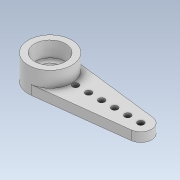
# Autodesk Inventor part: sg90舵盘01
Saved by Autodesk Inventor 2022.5 (Build 265521000, 521)
## iProperties
Created: 2024-03-17
Part Number: sg90舵盘01
Material: 常规
Document SubType Name: Modeling
Designer: Gagouking
Density: 1 g/cm^3
Appearance: 默认
Author: Gagouking
Autodesk Inventor part; units mm, degrees
ref_plane "YZ Plane" through (0, 0, 0) normal (1, 0, 0) x (0, 1, 0)
ref_plane "XZ Plane" through (0, 0, 0) normal (0, 1, 0) x (-1, 0, 0)
ref_plane "XY Plane" through (0, 0, 0) normal (0, 0, 1) x (1, 0, 0)
sketch "草图1" plane through (0, 0, 0) normal (0, 1, 0) x (-1, 0, 0)
  circle A0 centre (0, 0) radius 1.5
  line L0 (0, 0) -> (-13.1253, 0) construction
  circle A1 centre (-4.1, 0) radius 0.5
  circle A2 centre (-6.2, 0) radius 0.5
  circle A3 centre (-8.3, 0) radius 0.5
  circle A4 centre (-10.4, 0) radius 0.5
  circle A5 centre (-12.5, 0) radius 0.5
  circle A6 centre (-14.6, 0) radius 0.5
  arc A7 (-0.4195, -3.4748) -> (-0.4195, 3.4748) centre (0, 0) ccw
  arc A8 (-14.8098, 1.7374) -> (-14.8098, -1.7374) centre (-14.6, 0) ccw
  line L1 (-0.4195, -3.4748) -> (-14.8098, -1.7374)
  line L2 (-0.4195, 3.4748) -> (-14.8098, 1.7374)
  dimension "d0" = 3
  dimension "d1" = 1
  dimension "d2" = 4.1
  dimension "d5" = 2.1
  dimension "d10" = 7
  dimension "d11" = 3.5
  constraints: 9 centre point, 6 end point, 4 point on circle, 4 tangent, 3 coincident, 2 horizontal, 1 point on line, 10 other
  measures "d0" diameter of A0
  measures "d1" diameter of A1
  measures "d2" distance of point (0, 0) A1.centre
  measures "d5" distance of A1.centre A2.centre
  measures "d10" diameter of A7
  measures "d11" diameter of A8
extrude "拉伸1" add sketch "草图1" along normal blind 1.5
sketch "草图2" plane through (0, 1.5, 0) normal (0, 1, 0) x (1, 0, 0)
  circle A0 centre (0, 0) radius 3.5
  line L0 (0.4195, -3.4748) -> (14.8098, -1.7374) projected
  arc A1 (14.8098, -1.7374) -> (14.8098, 1.7374) centre (14.6, 0) ccw projected
  line L1 (14.8098, 1.7374) -> (0.4195, 3.4748) projected
  arc A2 (0.4195, 3.4748) -> (0.4195, -3.4748) centre (0, 0) ccw projected
  circle A3 centre (4.1, 0) radius 0.5 projected
  circle A4 centre (6.2, 0) radius 0.5 projected
  circle A5 centre (8.3, 0) radius 0.5 projected
  circle A6 centre (10.4, 0) radius 0.5 projected
  circle A7 centre (12.5, 0) radius 0.5 projected
  circle A8 centre (14.6, 0) radius 0.5 projected
  circle A9 centre (0, 0) radius 1.5 projected
  circle A10 centre (0, 0) radius 2.5
  dimension "d16" = 5
  constraints: 2 centre point, 2 coincident, 1 concentric
  measures "d16" diameter of A10
extrude "拉伸2" add sketch "草图2" along normal blind 2.5 contours A0
